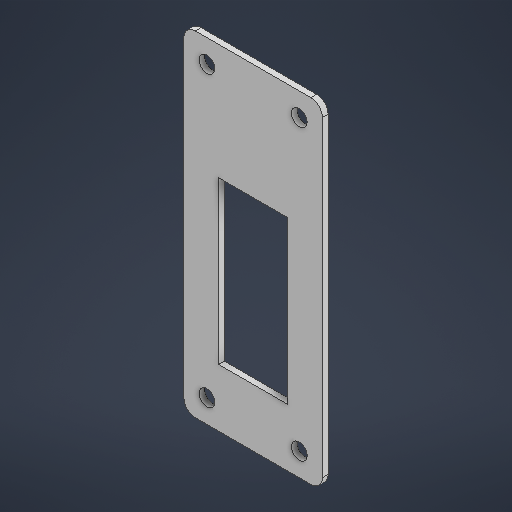
# Autodesk Inventor part: odompoly
Saved by Autodesk Inventor 2026.1 (Build 301233000, 233)
## iProperties
Created: 2026-03-12
Part Number: odompoly
Material: Generic
Document SubType Name: Modeling
Designer: roejo
Density: 1 g/cm^3
Appearance: Default
Author: roejo
Autodesk Inventor part; units mm, degrees
ref_plane "YZ Plane" through (0, 0, 0) normal (1, 0, 0) x (0, 1, 0)
ref_plane "XZ Plane" through (0, 0, 0) normal (0, 1, 0) x (-1, 0, 0)
ref_plane "XY Plane" through (0, 0, 0) normal (0, 0, 1) x (1, 0, 0)
sketch "Sketch1" plane through (0, 0, 0) normal (0, 0, 1) x (1, 0, 0)
  line L0 (3.175, 0) -> (34.925, 0)
  line L1 (38.1, 3.175) -> (38.1, 88.9)
  line L2 (34.925, 92.075) -> (3.175, 92.075)
  line L3 (0, 88.9) -> (0, 3.175)
  circle A0 centre (6.35, 85.725) radius 2.1844
  circle A1 centre (31.75, 85.725) radius 2.1844
  circle A2 centre (31.75, 6.35) radius 2.1844
  circle A3 centre (6.35, 6.35) radius 2.1844
  arc A4 (3.175, 92.075) -> (0, 88.9) centre (3.175, 88.9) ccw
  arc A5 (38.1, 88.9) -> (34.925, 92.075) centre (34.925, 88.9) ccw
  arc A6 (34.925, 0) -> (38.1, 3.175) centre (34.925, 3.175) ccw
  arc A7 (0, 3.175) -> (3.175, 0) centre (3.175, 3.175) ccw
  line L4 (9.525, 60.325) -> (28.575, 60.325)
  line L5 (28.575, 60.325) -> (28.575, 15.875)
  line L6 (28.575, 15.875) -> (9.525, 15.875)
  line L7 (9.525, 15.875) -> (9.525, 60.325)
  point P0 (0, 0)
  point P1 (38.1, 92.075)
  point P2 (38.1, 0)
  point P3 (0, 92.075)
  dimension "d0" = 38.1
  dimension "d1" = 92.075
  dimension "d2" = 4.3688
  dimension "d3" = 4.3688
  dimension "d4" = 4.3688
  dimension "d5" = 4.3688
  dimension "d6" = 0
  dimension "d7" = 25.4
  dimension "d8" = 0
  dimension "d9" = 79.375
  dimension "d10" = 0
  dimension "d11" = 79.375
  dimension "d12" = 6.35
  dimension "d13" = 6.35
  dimension "d14" = 3.175
  dimension "d16" = 25.4
  dimension "d17" = 9.525
  dimension "d18" = 9.525
  dimension "d19" = 9.525
  constraints: 16 end point, 8 centre point, 8 point on circle, 8 point on line, 8 tangent, 4 parallel, 3 equal radius, 2 horizontal, 2 perpendicular
  measures "d0" distance of point (0, 92.075) point (38.1, 92.075)
  measures "d1" distance of point (38.1, 92.075) point (38.1, 0)
  measures "d2" diameter of A0
  measures "d3" diameter of A1
  measures "d4" diameter of A2
  measures "d5" diameter of A3
  measures "d6" vertical distance of A1.centre A0.centre
  measures "d7" distance of A1.centre A0.centre
  measures "d8" horizontal distance of A3.centre A0.centre
  measures "d9" distance of A3.centre A0.centre
  measures "d10" horizontal distance of A1.centre A2.centre
  measures "d11" distance of A1.centre A2.centre
  measures "d12" distance from line of L1 A2.centre
  measures "d13" distance from line of L0 A2.centre
  measures "d14" radius of A4
  measures "d16" distance from line of A0.centre L4
  measures "d17" distance between parallel lines of L1 L5
  measures "d18" distance between parallel lines of L3 L7
  measures "d19" vertical distance of L6.end A3.centre
extrude "Extrusion1" add sketch "Sketch1" along normal blind 1.5875
body "Solid1"
